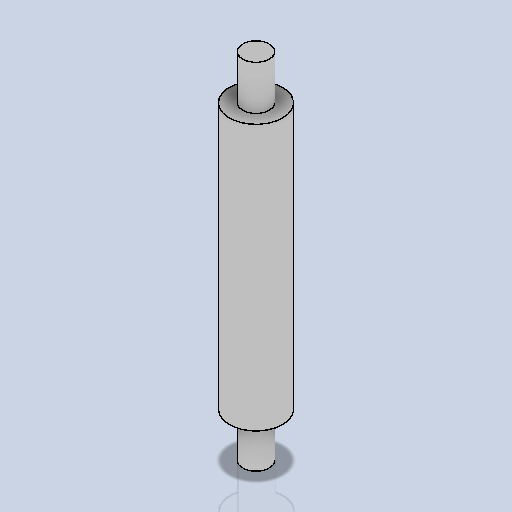
# Autodesk Inventor part: drum
Saved by Autodesk Inventor 2026.1 (Build 301233000, 233)
## iProperties
Created: 2025-08-31
Part Number: drum
Material: Generic
Document SubType Name: Modeling
Designer: baseb
Density: 1 g/cm^3
Appearance: Default
Author: baseb
Autodesk Inventor part; units mm, degrees
ref_plane "YZ Plane" through (0, 0, 0) normal (1, 0, 0) x (0, 1, 0)
ref_plane "XZ Plane" through (0, 0, 0) normal (0, 1, 0) x (-1, 0, 0)
ref_plane "XY Plane" through (0, 0, 0) normal (0, 0, 1) x (1, 0, 0)
sketch "Sketch1" plane through (0, 0, 0) normal (0, 1, 0) x (-1, 0, 0)
  circle A0 centre (0, 0) radius 9.525
  dimension "d0" = 19.05
  constraints: 1 centre point, 1 coincident
  measures "d0" diameter of A0
extrude "Extrusion1" add sketch "Sketch1" along normal mid plane 127
sketch "Sketch2" plane through (0, 63.5, 0) normal (0, 1, 0) x (1, 0, 0)
  circle A0 centre (0, 0) radius 9.525
  circle A1 centre (0, 0) radius 4.7625
  dimension "d3" = 9.525
  dimension "d4" = 19.05
  constraints: 2 centre point, 2 coincident
  measures "d3" diameter of A1
  measures "d4" diameter of A0
extrude "Extrusion2" cut sketch "Sketch2" against normal blind 15.875
sketch "Sketch3" plane through (0, -63.5, 0) normal (0, -1, 0) x (1, 0, 0)
  circle A0 centre (0, 0) radius 4.7625
  circle A1 centre (0, 0) radius 9.525
  dimension "d7" = 9.525
  constraints: 2 centre point, 2 coincident
  measures "d7" diameter of A0
extrude "Extrusion3" cut sketch "Sketch3" against normal blind 15.875
body "Solid1"
